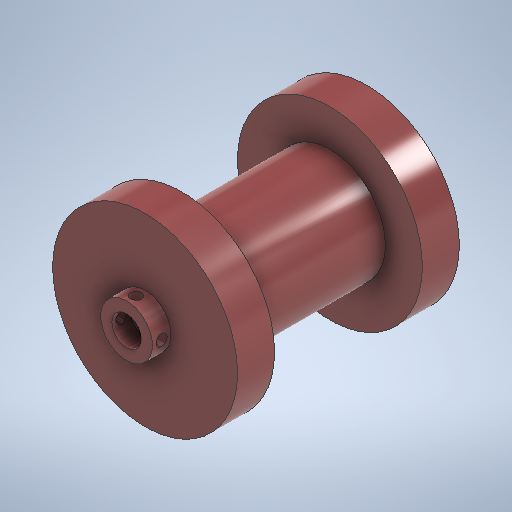
# Autodesk Inventor part: carrete_V1
Saved by Autodesk Inventor 2026 (Build 300175050, 175E)
## iProperties
Created: 2025-06-24
Part Number: carrete_V1
Material: Genérico
Document SubType Name: Modeling
Designer: piero
Density: 1 g/cm^3
Appearance: Valor por defecto
Author: piero
Autodesk Inventor part; units mm, degrees
ref_plane "YZ Plane" through (0, 0, 0) normal (1, 0, 0) x (0, 1, 0)
ref_plane "XZ Plane" through (0, 0, 0) normal (0, 1, 0) x (-1, 0, 0)
ref_plane "XY Plane" through (0, 0, 0) normal (0, 0, 1) x (1, 0, 0)
sketch "Boceto1" plane through (0, 0, 0) normal (0, 0, 1) x (1, 0, 0)
  circle A0 centre (0, 0) radius 25
  circle A1 centre (0, 0) radius 4
  circle A2 centre (0, 0) radius 11
  dimension "d0" = 50
  dimension "d3" = 8
  dimension "d34" = 22
  constraints: 3 centre point, 3 coincident
  measures "d0" diameter of A0
  measures "d3" diameter of A1
  measures "d34" diameter of A2
extrude "Extrusión1" add sketch "Boceto1" along normal blind 10 contours A0 | A2
sketch "Boceto5" plane through (0, 0, 10) normal (0, 0, 1) x (1, 0, 0)
  circle A0 centre (0, 0) radius 5
  circle A1 centre (0, 0) radius 15
  dimension "d15" = 10
  dimension "d16" = 30
  constraints: 2 centre point, 2 coincident
  measures "d15" diameter of A0
  measures "d16" diameter of A1
extrude "Extrusión5" add sketch "Boceto5" along normal blind 40
sketch "Boceto6" plane through (0, 0, 50) normal (0, 0, 1) x (1, 0, 0)
  circle A0 centre (0, 0) radius 4 projected
  circle A1 centre (0, 0) radius 25
  circle A2 centre (0, 0) radius 4
  circle A3 centre (0, 0) radius 5 projected
  circle A4 centre (0, 0) radius 11
  dimension "d22" = 50
  dimension "d30" = 8
  dimension "d31" = 22
  constraints: 3 centre point, 2 coincident
  measures "d22" diameter of A1
  measures "d30" diameter of A2
  measures "d31" diameter of A4
extrude "Extrusión6" add sketch "Boceto6" along normal blind 10 contours A1 | A4
sketch "Boceto10" plane through (0, 0, 60) normal (0, 0, 1) x (1, 0, 0)
  circle A0 centre (0, 0) radius 7
  circle A1 centre (0, 0) radius 4
  dimension "d41" = 14
  dimension "d42" = 8
  constraints: 2 centre point, 2 coincident
  measures "d41" diameter of A0
  measures "d42" diameter of A1
extrude "Extrusión11" add sketch "Boceto10" along normal blind 5
sketch "Boceto11" plane through (0, 0, 0) normal (0, 0, -1) x (-1, 0, 0)
  circle A0 centre (0, 0) radius 4
  circle A1 centre (0, 0) radius 7
  dimension "d45" = 8
  dimension "d46" = 14
  constraints: 2 centre point, 2 coincident
  measures "d45" diameter of A0
  measures "d46" diameter of A1
extrude "Extrusión12" add sketch "Boceto11" along normal blind 5
sketch "Boceto12" plane through (0, 0, 0) normal (1, 0, 0) x (0, 1, 0)
  circle A0 centre (0, 62.5) radius 1.5
  circle A1 centre (0, -2.5056) radius 1.5
  point P0 (0, 0)
  dimension "d49" = 3
  dimension "d50" = 3
  constraints: 2 centre point
  measures "d49" diameter of A0
  measures "d50" diameter of A1
hole "Agujero1" at (0, 0, 62.5) direction (-1, 0, 0) diameter 3 end through all
sketch "Boceto13" plane through (0, 0, 0) normal (0, 1, 0) x (-1, 0, 0)
  circle A0 centre (0, 62.4533) radius 1.5
  circle A1 centre (0, -2.49) radius 1.5
  point P0 (0, 0)
  dimension "d58" = 3
  dimension "d59" = 3
  constraints: 2 centre point
  measures "d58" diameter of A0
  measures "d59" diameter of A1
hole "Agujero2" at (0, 0, -2.49) direction (0, 1, 0) diameter 3 end through all
sketch "Boceto14" plane through (0, 0, 0) normal (1, 0, 0) x (0, 1, 0)
  circle A0 centre (0, 62.5132) radius 1.5
  circle A1 centre (0, -2.3779) radius 1.5
  point P0 (0, 0)
  dimension "d67" = 3
  dimension "d68" = 3
  constraints: 2 centre point
  measures "d67" diameter of A0
  measures "d68" diameter of A1
hole "Agujero3" at (0, 0, 62.5132) direction (1, 0, 0) diameter 3 end through all
hole "Agujero4" at (0, 0, -2.3779) direction (-1, 0, 0) diameter 3 end through all
sketch "Boceto15" plane through (0, 0, 0) normal (1, 0, 0) x (0, 1, 0)
  circle A0 centre (0, -2.3219) radius 1.5
  point P0 (0, 0)
  dimension "d83" = 3
  constraints: 1 centre point
  measures "d83" diameter of A0
hole "Agujero5" at (0, 0, -2.3219) direction (1, 0, 0) diameter 3 end through all
sketch "Boceto16" plane through (0, 0, 0) normal (0, 1, 0) x (-1, 0, 0)
  circle A0 centre (0, 62.5122) radius 1.5
  point P0 (0, 0)
  dimension "d91" = 3
  constraints: 1 centre point
  measures "d91" diameter of A0
hole "Agujero6" at (0, 0, 62.5122) direction (0, 1, 0) diameter 3 end through all
